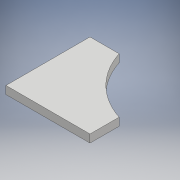
# Autodesk Inventor part: Naroznik_54x54
Saved by Autodesk Inventor 2018 (Build 220112000, 112)
## iProperties
Created: 2018-10-19
Part Number: Naroznik_54x54
Material: Ogólny
Document SubType Name: Modeling
Designer: EWA
Density: 1 g/cm^3
Appearance: Domyślna
Author: EWA
Autodesk Inventor part; units mm, degrees
ref_plane "YZ Plane" through (0, 0, 0) normal (1, 0, 0) x (0, 1, 0)
ref_plane "XZ Plane" through (0, 0, 0) normal (0, 1, 0) x (-1, 0, 0)
ref_plane "XY Plane" through (0, 0, 0) normal (0, 0, 1) x (1, 0, 0)
sketch "Szkic1" plane through (0, 0, 0) normal (0, 0, 1) x (1, 0, 0)
  line L0 (0, 0) -> (64, 0) construction
  line L1 (64, 0) -> (64, 64) construction
  line L2 (64, 64) -> (0, 64) construction
  line L3 (0, 64) -> (0, 0) construction
  line L4 (0, 0) -> (168, 0) construction
  line L5 (168, 0) -> (168, 168) construction
  line L6 (168, 168) -> (0, 168) construction
  line L7 (0, 168) -> (0, 0) construction
  line L8 (84, 168) -> (84, 0) construction
  circle A0 centre (84, 84) radius 65 construction
  line L9 (0, 0) -> (64, 0)
  line L10 (64, 0) -> (64, 22.1534)
  line L11 (0, 0) -> (0, 64)
  line L12 (0, 64) -> (22.1534, 64)
  arc A1 (22.1534, 64) -> (64, 22.1534) centre (84, 84) ccw
  dimension "d7" = 64
  dimension "d8" = 64
  dimension "d9" = 168
  dimension "d10" = 168
  dimension "d11" = 130
  dimension "d12" = 64
  dimension "d13" = 64
  constraints: 26 end point, 4 parallel, 4 point on circle, 3 collinear, 3 midpoint, 3 perpendicular, 2 centre point, 2 horizontal, 2 point on line, 1 concentric
  measures "d7" distance of L2.end L1.end
  measures "d8" distance of L1.end L0.end
  measures "d9" distance of L6.end L5.end
  measures "d10" distance of L5.end L4.end
  measures "d11" diameter of A0
  measures "d12" distance of L0.start L0.end
  measures "d13" distance of L0.start L2.end
extrude "Wyciągnięcie proste1" add sketch "Szkic1" along normal blind 6
equation "\"d7\" = d8"
